Autodesk Fusion 360 part; units mm, degrees
(part 2 of 2)
  spline S17 degree 5 poles (16.2711, -4.6208) (16.2922, -4.6268) (16.3347, -4.6379) (16.399, -4.6517) (16.4857, -4.6647) (16.5954, -4.6738) (16.706, -4.6779) (16.8173, -4.6789) (16.9288, -4.6784) (17.0405, -4.6766) (17.1524, -4.6734) (17.2646, -4.6683) (17.377, -4.6608) (17.4898, -4.6505) (17.6029, -4.6377) (17.7161, -4.6224) (17.8296, -4.6052) (17.9431, -4.5863) (18.0567, -4.5658) (18.1703, -4.5438) (18.284, -4.5203) (18.3977, -4.4951) (18.5115, -4.4682) (18.6252, -4.4395) (18.739, -4.4092) (18.8527, -4.3772) (18.9664, -4.3437) (19.08, -4.3087) (19.1936, -4.2723) (19.3071, -4.2345) (19.4204, -4.1952) (19.5337, -4.1545) (19.6469, -4.1124) (19.7599, -4.0688) (19.8727, -4.0239) (19.9855, -3.9776) (20.098, -3.9299) (20.2104, -3.8809) (20.3225, -3.8306) (20.4345, -3.779) (20.5463, -3.7261) (20.6578, -3.6719) (20.7692, -3.6164) (20.8802, -3.5597) (20.9911, -3.5017) (21.1017, -3.4425) (21.212, -3.3821) (21.322, -3.3204) (21.4317, -3.2575) (21.5412, -3.1935) (21.6503, -3.1282) (21.7592, -3.0618) (21.8677, -2.9942) (21.9759, -2.9255) (22.0837, -2.8556) (22.1912, -2.7845) (22.2984, -2.7123) (22.4052, -2.639) (22.5116, -2.5646) (22.6176, -2.4891) (22.7233, -2.4125) (22.8286, -2.3348) (22.9335, -2.256) (23.0379, -2.1761) (23.142, -2.0952) (23.2456, -2.0132) (23.3488, -1.9301) (23.4516, -1.846) (23.5539, -1.7609) (23.6558, -1.6748) (23.7572, -1.5876) (23.838, -1.517) (23.8983, -1.4636) (23.9385, -1.4279) (23.9586, -1.4099) knots 0 0 0 0 0 0 0.01428571 0.02857143 0.04285714 0.05714286 0.07142857 0.08571429 0.1 0.11428571 0.12857143 0.14285714 0.15714286 0.17142857 0.18571429 0.2 0.21428571 0.22857143 0.24285714 0.25714286 0.27142857 0.28571429 0.3 0.31428571 0.32857143 0.34285714 0.35714286 0.37142857 0.38571429 0.4 0.41428571 0.42857143 0.44285714 0.45714286 0.47142857 0.48571429 0.5 0.51428571 0.52857143 0.54285714 0.55714286 0.57142857 0.58571429 0.6 0.61428571 0.62857143 0.64285714 0.65714286 0.67142857 0.68571429 0.7 0.71428571 0.72857143 0.74285714 0.75714286 0.77142857 0.78571429 0.8 0.81428571 0.82857143 0.84285714 0.85714286 0.87142857 0.88571429 0.9 0.91428571 0.92857143 0.94285714 0.95714286 0.97142857 0.98571429 1 1 1 1 1 1
  spline S18 degree 5 poles (-12.1373, -11.7808) (-12.1531, -11.7961) (-12.1839, -11.8274) (-12.228, -11.8761) (-12.2826, -11.9447) (-12.3454, -12.0351) (-12.4042, -12.1289) (-12.4607, -12.2247) (-12.516, -12.3216) (-12.5703, -12.4192) (-12.6235, -12.5177) (-12.6752, -12.6174) (-12.7249, -12.7185) (-12.7724, -12.8213) (-12.8178, -12.9257) (-12.8612, -13.0314) (-12.903, -13.1383) (-12.9434, -13.2461) (-12.9825, -13.3547) (-13.0203, -13.4641) (-13.0567, -13.5743) (-13.0917, -13.6853) (-13.1253, -13.7973) (-13.1573, -13.9101) (-13.1879, -14.0238) (-13.2171, -14.1383) (-13.245, -14.2535) (-13.2715, -14.3694) (-13.2967, -14.486) (-13.3207, -14.6032) (-13.3434, -14.721) (-13.3648, -14.8394) (-13.3849, -14.9585) (-13.4037, -15.0781) (-13.4212, -15.1983) (-13.4374, -15.3191) (-13.4524, -15.4404) (-13.4661, -15.5622) (-13.4787, -15.6845) (-13.49, -15.8073) (-13.5, -15.9306) (-13.5089, -16.0543) (-13.5165, -16.1784) (-13.5229, -16.303) (-13.5281, -16.4279) (-13.5321, -16.5533) (-13.5349, -16.6791) (-13.5365, -16.8052) (-13.537, -16.9317) (-13.5362, -17.0585) (-13.5343, -17.1856) (-13.5312, -17.3131) (-13.5269, -17.4409) (-13.5215, -17.5689) (-13.5148, -17.6973) (-13.5071, -17.8259) (-13.4981, -17.9548) (-13.4881, -18.0839) (-13.4768, -18.2133) (-13.4644, -18.3429) (-13.4509, -18.4727) (-13.4363, -18.6027) (-13.4205, -18.733) (-13.4035, -18.8634) (-13.3855, -18.994) (-13.3663, -19.1247) (-13.3459, -19.2556) (-13.3245, -19.3866) (-13.3019, -19.5178) (-13.2783, -19.6491) (-13.2535, -19.7805) (-13.2328, -19.8858) (-13.2167, -19.9647) (-13.2058, -20.0174) (-13.2003, -20.0438) knots 0 0 0 0 0 0 0.01428571 0.02857143 0.04285714 0.05714286 0.07142857 0.08571429 0.1 0.11428571 0.12857143 0.14285714 0.15714286 0.17142857 0.18571429 0.2 0.21428571 0.22857143 0.24285714 0.25714286 0.27142857 0.28571429 0.3 0.31428571 0.32857143 0.34285714 0.35714286 0.37142857 0.38571429 0.4 0.41428571 0.42857143 0.44285714 0.45714286 0.47142857 0.48571429 0.5 0.51428571 0.52857143 0.54285714 0.55714286 0.57142857 0.58571429 0.6 0.61428571 0.62857143 0.64285714 0.65714286 0.67142857 0.68571429 0.7 0.71428571 0.72857143 0.74285714 0.75714286 0.77142857 0.78571429 0.8 0.81428571 0.82857143 0.84285714 0.85714286 0.87142857 0.88571429 0.9 0.91428571 0.92857143 0.94285714 0.95714286 0.97142857 0.98571429 1 1 1 1 1 1
  spline S19 degree 5 poles (-13.2003, 20.0438) (-13.2058, 20.0174) (-13.2167, 19.9647) (-13.2328, 19.8858) (-13.2535, 19.7805) (-13.2783, 19.6491) (-13.3019, 19.5178) (-13.3245, 19.3866) (-13.3459, 19.2556) (-13.3663, 19.1247) (-13.3855, 18.994) (-13.4035, 18.8634) (-13.4205, 18.733) (-13.4363, 18.6027) (-13.4509, 18.4727) (-13.4644, 18.3429) (-13.4768, 18.2133) (-13.4881, 18.0839) (-13.4981, 17.9548) (-13.5071, 17.8259) (-13.5148, 17.6973) (-13.5215, 17.5689) (-13.5269, 17.4409) (-13.5312, 17.3131) (-13.5343, 17.1856) (-13.5362, 17.0585) (-13.537, 16.9317) (-13.5365, 16.8052) (-13.5349, 16.6791) (-13.5321, 16.5533) (-13.5281, 16.4279) (-13.5229, 16.303) (-13.5165, 16.1784) (-13.5089, 16.0543) (-13.5, 15.9306) (-13.49, 15.8073) (-13.4787, 15.6845) (-13.4661, 15.5622) (-13.4524, 15.4404) (-13.4374, 15.3191) (-13.4212, 15.1983) (-13.4037, 15.0781) (-13.3849, 14.9585) (-13.3648, 14.8394) (-13.3434, 14.721) (-13.3207, 14.6032) (-13.2967, 14.486) (-13.2715, 14.3694) (-13.245, 14.2535) (-13.2171, 14.1383) (-13.1879, 14.0238) (-13.1573, 13.9101) (-13.1253, 13.7973) (-13.0917, 13.6853) (-13.0567, 13.5743) (-13.0203, 13.4641) (-12.9825, 13.3547) (-12.9434, 13.2461) (-12.903, 13.1383) (-12.8612, 13.0314) (-12.8178, 12.9257) (-12.7724, 12.8213) (-12.7249, 12.7185) (-12.6752, 12.6174) (-12.6235, 12.5177) (-12.5703, 12.4192) (-12.516, 12.3216) (-12.4607, 12.2247) (-12.4042, 12.1289) (-12.3454, 12.0351) (-12.2826, 11.9447) (-12.228, 11.8761) (-12.1839, 11.8274) (-12.1531, 11.7961) (-12.1373, 11.7808) knots -1 -1 -1 -1 -1 -1 -0.98571429 -0.97142857 -0.95714286 -0.94285714 -0.92857143 -0.91428571 -0.9 -0.88571429 -0.87142857 -0.85714286 -0.84285714 -0.82857143 -0.81428571 -0.8 -0.78571429 -0.77142857 -0.75714286 -0.74285714 -0.72857143 -0.71428571 -0.7 -0.68571429 -0.67142857 -0.65714286 -0.64285714 -0.62857143 -0.61428571 -0.6 -0.58571429 -0.57142857 -0.55714286 -0.54285714 -0.52857143 -0.51428571 -0.5 -0.48571429 -0.47142857 -0.45714286 -0.44285714 -0.42857143 -0.41428571 -0.4 -0.38571429 -0.37142857 -0.35714286 -0.34285714 -0.32857143 -0.31428571 -0.3 -0.28571429 -0.27142857 -0.25714286 -0.24285714 -0.22857143 -0.21428571 -0.2 -0.18571429 -0.17142857 -0.15714286 -0.14285714 -0.12857143 -0.11428571 -0.1 -0.08571429 -0.07142857 -0.05714286 -0.04285714 -0.02857143 -0.01428571 0 0 0 0 0 0
  arc A49 (10.7583, -21.4537) -> (13.2003, -20.0438) centre (0, 0) ccw
  arc A50 (-3.1536, 12.5126) -> (-1.0283, 11.0101) centre (-1.2143, 13.0014) ccw
  spline S20 degree 5 poles (4.1338, -16.4016) (4.1392, -16.4229) (4.1508, -16.4652) (4.171, -16.5278) (4.2031, -16.6094) (4.25, -16.709) (4.3019, -16.8068) (4.3566, -16.9036) (4.4128, -16.9999) (4.4702, -17.0958) (4.5289, -17.1911) (4.5894, -17.2857) (4.6521, -17.3793) (4.7174, -17.4719) (4.7851, -17.5634) (4.8549, -17.6538) (4.9266, -17.7435) (4.9997, -17.8323) (5.0742, -17.9205) (5.1501, -18.0079) (5.2273, -18.0946) (5.306, -18.1804) (5.3862, -18.2655) (5.4679, -18.3497) (5.551, -18.433) (5.6356, -18.5155) (5.7214, -18.5972) (5.8085, -18.6782) (5.8969, -18.7583) (5.9864, -18.8377) (6.0771, -18.9162) (6.1689, -18.9939) (6.262, -19.0709) (6.3562, -19.147) (6.4516, -19.2222) (6.548, -19.2967) (6.6456, -19.3703) (6.7442, -19.4431) (6.8439, -19.5151) (6.9446, -19.5863) (7.0463, -19.6567) (7.149, -19.7262) (7.2527, -19.7948) (7.3573, -19.8627) (7.463, -19.9297) (7.5695, -19.9958) (7.677, -20.0611) (7.7854, -20.1256) (7.8948, -20.1892) (8.005, -20.2519) (8.116, -20.3138) (8.228, -20.3749) (8.3408, -20.4351) (8.4544, -20.4944) (8.5689, -20.5528) (8.6842, -20.6104) (8.8002, -20.6671) (8.9171, -20.723) (9.0348, -20.7779) (9.1532, -20.832) (9.2724, -20.8852) (9.3923, -20.9375) (9.513, -20.9889) (9.6344, -21.0395) (9.7565, -21.0891) (9.8794, -21.1379) (10.0029, -21.1857) (10.1271, -21.2327) (10.252, -21.2787) (10.3775, -21.3239) (10.5037, -21.3681) (10.6052, -21.4028) (10.6816, -21.4284) (10.7327, -21.4453) (10.7583, -21.4537) knots 0 0 0 0 0 0 0.01428571 0.02857143 0.04285714 0.05714286 0.07142857 0.08571429 0.1 0.11428571 0.12857143 0.14285714 0.15714286 0.17142857 0.18571429 0.2 0.21428571 0.22857143 0.24285714 0.25714286 0.27142857 0.28571429 0.3 0.31428571 0.32857143 0.34285714 0.35714286 0.37142857 0.38571429 0.4 0.41428571 0.42857143 0.44285714 0.45714286 0.47142857 0.48571429 0.5 0.51428571 0.52857143 0.54285714 0.55714286 0.57142857 0.58571429 0.6 0.61428571 0.62857143 0.64285714 0.65714286 0.67142857 0.68571429 0.7 0.71428571 0.72857143 0.74285714 0.75714286 0.77142857 0.78571429 0.8 0.81428571 0.82857143 0.84285714 0.85714286 0.87142857 0.88571429 0.9 0.91428571 0.92857143 0.94285714 0.95714286 0.97142857 0.98571429 1 1 1 1 1 1
  spline S21 degree 5 poles (-23.9586, -1.4099) (-23.9385, -1.4279) (-23.8983, -1.4636) (-23.838, -1.517) (-23.7572, -1.5876) (-23.6558, -1.6748) (-23.5539, -1.7609) (-23.4516, -1.846) (-23.3488, -1.9301) (-23.2456, -2.0132) (-23.142, -2.0952) (-23.0379, -2.1761) (-22.9335, -2.256) (-22.8286, -2.3348) (-22.7233, -2.4125) (-22.6176, -2.4891) (-22.5116, -2.5646) (-22.4052, -2.639) (-22.2984, -2.7123) (-22.1912, -2.7845) (-22.0837, -2.8556) (-21.9759, -2.9255) (-21.8677, -2.9942) (-21.7592, -3.0618) (-21.6503, -3.1282) (-21.5412, -3.1935) (-21.4317, -3.2575) (-21.322, -3.3204) (-21.212, -3.3821) (-21.1017, -3.4425) (-20.9911, -3.5017) (-20.8802, -3.5597) (-20.7692, -3.6164) (-20.6578, -3.6719) (-20.5463, -3.7261) (-20.4345, -3.779) (-20.3225, -3.8306) (-20.2104, -3.8809) (-20.098, -3.9299) (-19.9855, -3.9776) (-19.8727, -4.0239) (-19.7599, -4.0688) (-19.6469, -4.1124) (-19.5337, -4.1545) (-19.4204, -4.1952) (-19.3071, -4.2345) (-19.1936, -4.2723) (-19.08, -4.3087) (-18.9664, -4.3437) (-18.8527, -4.3772) (-18.739, -4.4092) (-18.6252, -4.4395) (-18.5115, -4.4682) (-18.3977, -4.4951) (-18.284, -4.5203) (-18.1703, -4.5438) (-18.0567, -4.5658) (-17.9431, -4.5863) (-17.8296, -4.6052) (-17.7161, -4.6224) (-17.6029, -4.6377) (-17.4898, -4.6505) (-17.377, -4.6608) (-17.2646, -4.6683) (-17.1524, -4.6734) (-17.0405, -4.6766) (-16.9288, -4.6784) (-16.8173, -4.6789) (-16.706, -4.6779) (-16.5954, -4.6738) (-16.4857, -4.6647) (-16.399, -4.6517) (-16.3347, -4.6379) (-16.2922, -4.6268) (-16.2711, -4.6208) knots -1 -1 -1 -1 -1 -1 -0.98571429 -0.97142857 -0.95714286 -0.94285714 -0.92857143 -0.91428571 -0.9 -0.88571429 -0.87142857 -0.85714286 -0.84285714 -0.82857143 -0.81428571 -0.8 -0.78571429 -0.77142857 -0.75714286 -0.74285714 -0.72857143 -0.71428571 -0.7 -0.68571429 -0.67142857 -0.65714286 -0.64285714 -0.62857143 -0.61428571 -0.6 -0.58571429 -0.57142857 -0.55714286 -0.54285714 -0.52857143 -0.51428571 -0.5 -0.48571429 -0.47142857 -0.45714286 -0.44285714 -0.42857143 -0.41428571 -0.4 -0.38571429 -0.37142857 -0.35714286 -0.34285714 -0.32857143 -0.31428571 -0.3 -0.28571429 -0.27142857 -0.25714286 -0.24285714 -0.22857143 -0.21428571 -0.2 -0.18571429 -0.17142857 -0.15714286 -0.14285714 -0.12857143 -0.11428571 -0.1 -0.08571429 -0.07142857 -0.05714286 -0.04285714 -0.02857143 -0.01428571 0 0 0 0 0 0
  spline S22 degree 5 poles (-4.1338, 16.4016) (-4.1392, 16.4229) (-4.1508, 16.4652) (-4.171, 16.5278) (-4.2031, 16.6094) (-4.25, 16.709) (-4.3019, 16.8068) (-4.3566, 16.9036) (-4.4128, 16.9999) (-4.4702, 17.0958) (-4.5289, 17.1911) (-4.5894, 17.2857) (-4.6521, 17.3793) (-4.7174, 17.4719) (-4.7851, 17.5634) (-4.8549, 17.6538) (-4.9266, 17.7435) (-4.9997, 17.8323) (-5.0742, 17.9205) (-5.1501, 18.0079) (-5.2273, 18.0946) (-5.306, 18.1804) (-5.3862, 18.2655) (-5.4679, 18.3497) (-5.551, 18.433) (-5.6356, 18.5155) (-5.7214, 18.5972) (-5.8085, 18.6782) (-5.8969, 18.7583) (-5.9864, 18.8377) (-6.0771, 18.9162) (-6.1689, 18.9939) (-6.262, 19.0709) (-6.3562, 19.147) (-6.4516, 19.2222) (-6.548, 19.2967) (-6.6456, 19.3703) (-6.7442, 19.4431) (-6.8439, 19.5151) (-6.9446, 19.5863) (-7.0463, 19.6567) (-7.149, 19.7262) (-7.2527, 19.7948) (-7.3573, 19.8627) (-7.463, 19.9297) (-7.5695, 19.9958) (-7.677, 20.0611) (-7.7854, 20.1256) (-7.8948, 20.1892) (-8.005, 20.2519) (-8.116, 20.3138) (-8.228, 20.3749) (-8.3408, 20.4351) (-8.4544, 20.4944) (-8.5689, 20.5528) (-8.6842, 20.6104) (-8.8002, 20.6671) (-8.9171, 20.723) (-9.0348, 20.7779) (-9.1532, 20.832) (-9.2724, 20.8852) (-9.3923, 20.9375) (-9.513, 20.9889) (-9.6344, 21.0395) (-9.7565, 21.0891) (-9.8794, 21.1379) (-10.0029, 21.1857) (-10.1271, 21.2327) (-10.252, 21.2787) (-10.3775, 21.3239) (-10.5037, 21.3681) (-10.6052, 21.4028) (-10.6816, 21.4284) (-10.7327, 21.4453) (-10.7583, 21.4537) knots 0 0 0 0 0 0 0.01428571 0.02857143 0.04285714 0.05714286 0.07142857 0.08571429 0.1 0.11428571 0.12857143 0.14285714 0.15714286 0.17142857 0.18571429 0.2 0.21428571 0.22857143 0.24285714 0.25714286 0.27142857 0.28571429 0.3 0.31428571 0.32857143 0.34285714 0.35714286 0.37142857 0.38571429 0.4 0.41428571 0.42857143 0.44285714 0.45714286 0.47142857 0.48571429 0.5 0.51428571 0.52857143 0.54285714 0.55714286 0.57142857 0.58571429 0.6 0.61428571 0.62857143 0.64285714 0.65714286 0.67142857 0.68571429 0.7 0.71428571 0.72857143 0.74285714 0.75714286 0.77142857 0.78571429 0.8 0.81428571 0.82857143 0.84285714 0.85714286 0.87142857 0.88571429 0.9 0.91428571 0.92857143 0.94285714 0.95714286 0.97142857 0.98571429 1 1 1 1 1 1
  line L23 (12.4131, -3.5252) -> (16.2711, -4.6208)
  spline S23 degree 5 poles (-16.2711, 4.6208) (-16.2922, 4.6268) (-16.3347, 4.6379) (-16.399, 4.6517) (-16.4857, 4.6647) (-16.5954, 4.6738) (-16.706, 4.6779) (-16.8173, 4.6789) (-16.9288, 4.6784) (-17.0405, 4.6766) (-17.1524, 4.6734) (-17.2646, 4.6683) (-17.377, 4.6608) (-17.4898, 4.6505) (-17.6029, 4.6377) (-17.7161, 4.6224) (-17.8296, 4.6052) (-17.9431, 4.5863) (-18.0567, 4.5658) (-18.1703, 4.5438) (-18.284, 4.5203) (-18.3977, 4.4951) (-18.5115, 4.4682) (-18.6252, 4.4395) (-18.739, 4.4092) (-18.8527, 4.3772) (-18.9664, 4.3437) (-19.08, 4.3087) (-19.1936, 4.2723) (-19.3071, 4.2345) (-19.4204, 4.1952) (-19.5337, 4.1545) (-19.6469, 4.1124) (-19.7599, 4.0688) (-19.8727, 4.0239) (-19.9855, 3.9776) (-20.098, 3.9299) (-20.2104, 3.8809) (-20.3225, 3.8306) (-20.4345, 3.779) (-20.5463, 3.7261) (-20.6578, 3.6719) (-20.7692, 3.6164) (-20.8802, 3.5597) (-20.9911, 3.5017) (-21.1017, 3.4425) (-21.212, 3.3821) (-21.322, 3.3204) (-21.4317, 3.2575) (-21.5412, 3.1935) (-21.6503, 3.1282) (-21.7592, 3.0618) (-21.8677, 2.9942) (-21.9759, 2.9255) (-22.0837, 2.8556) (-22.1912, 2.7845) (-22.2984, 2.7123) (-22.4052, 2.639) (-22.5116, 2.5646) (-22.6176, 2.4891) (-22.7233, 2.4125) (-22.8286, 2.3348) (-22.9335, 2.256) (-23.0379, 2.1761) (-23.142, 2.0952) (-23.2456, 2.0132) (-23.3488, 1.9301) (-23.4516, 1.846) (-23.5539, 1.7609) (-23.6558, 1.6748) (-23.7572, 1.5876) (-23.838, 1.517) (-23.8983, 1.4636) (-23.9385, 1.4279) (-23.9586, 1.4099) knots 0 0 0 0 0 0 0.01428571 0.02857143 0.04285714 0.05714286 0.07142857 0.08571429 0.1 0.11428571 0.12857143 0.14285714 0.15714286 0.17142857 0.18571429 0.2 0.21428571 0.22857143 0.24285714 0.25714286 0.27142857 0.28571429 0.3 0.31428571 0.32857143 0.34285714 0.35714286 0.37142857 0.38571429 0.4 0.41428571 0.42857143 0.44285714 0.45714286 0.47142857 0.48571429 0.5 0.51428571 0.52857143 0.54285714 0.55714286 0.57142857 0.58571429 0.6 0.61428571 0.62857143 0.64285714 0.65714286 0.67142857 0.68571429 0.7 0.71428571 0.72857143 0.74285714 0.75714286 0.77142857 0.78571429 0.8 0.81428571 0.82857143 0.84285714 0.85714286 0.87142857 0.88571429 0.9 0.91428571 0.92857143 0.94285714 0.95714286 0.97142857 0.98571429 1 1 1 1 1 1
  arc A51 (9.0209, -6.3956) -> (9.2594, -8.9875) centre (10.6524, -7.5523) ccw
  arc A52 (-1.0283, -11.0101) -> (1.0283, -11.0101) centre (0, 0) ccw
extrude "Extrude3" add sketch "Spacer and Cap" along normal blind 4.2 separate body contours A24 A34 | A36 makes body 2
extrude "Extrude4" add sketch "Spacer and Cap" along normal blind 4.2 separate body contours A37 makes body 3
extrude "Extrude5" add 1 faces at (-8.6071, 0.7949, 8.4) along direction (0, 0, 1) blind 4.2 separate body on bodies 3 makes body 4
sketch "Motor attachment piece" plane through (0, 0, 12.6) normal (0, 0, 1) x (-1, 0, 0)
  circle A0 centre (0, 0) radius 10
  circle A1 centre (0, 0) radius 10
  circle A2 centre (0, 0) radius 2.7
  line L0 (1.85, -4) -> (-1.85, -4)
  line L1 (-1.85, -4) -> (-1.85, 4)
  line L2 (-1.85, 4) -> (1.85, 4)
  line L3 (1.85, 4) -> (1.85, -4)
  line L4 (1.85, -4) -> (-1.85, 4) construction
  line L5 (-1.85, -4) -> (1.85, 4) construction
  dimension "d16" = 5.4
  dimension "d17" = 3.7
  dimension "d18" = 8
  constraint horizontal L0
  constraint perpendicular L0 L1
  constraint parallel L0 L2
  constraint parallel L1 L3
  constraint coincident L4 A0.centre
  constraint coincident L5 A0.centre
  constraint coincident A0.centre A1.centre
  measures "d16" diameter of A2
  measures "d17" distance of L1.end L2.end
  measures "d18" distance of L0.end L1.end
extrude "Extrude6" add sketch "Motor attachment piece" along normal blind 4.2 separate body contours A0 A1 | A2 L3 | A2 L1 L2 L3 | A2 L0 L1 L3 | A2 L1 makes body 5
copy_body "CopyPasteBodies1" bodies 2 makes body 6
move_body "Move1" bodies 6 to x (1, 0, 0) y (0, 1, 0) z (0, 0, 1) at (-37.381, -1.1074, 0)
sketch "Back Cap" plane through (0, 0, 8.4) normal (0, 0, 1) x (-1, 0, 0)
  circle A0 centre (37.381, 1.1074) radius 3.25
  circle A1 centre (37.381, 1.1074) radius 6
  dimension "d23" = 12
  constraint concentric A0 A1
  measures "d23" diameter of A1
extrude "Extrude8" add sketch "Back Cap" against normal blind 4.2 bodies 6
move_body "Move2" bodies 3 to x (1, 0, 0) y (0, 1, 0) z (0, 0, 1) at (45.3922, 3.4121, 0)
move_body "Move3" bodies 4 to x (1, 0, 0) y (0, 1, 0) z (0, 0, 1) at (31.6318, -22.3587, 0)
move_body "Move4" bodies 2 to x (1, 0, 0) y (0, 1, 0) z (0, 0, 1) at (34.427, 25.1789, 0)
move_body "Move5" bodies 5 to x (1, 0, 0) y (0, 1, 0) z (0, 0, 1) at (-28.8671, -19.0156, 0)
move_body "Move6" bodies 3 to x (1, 0, 0) y (0, 1, 0) z (0, 0, 1) at (-76.3852, 16.0977, 0)
move_body "Move7" bodies 4 to x (1, 0, 0) y (0, 1, 0) z (0, 0, 1) at (-36.2987, 58.8671, 0)
move_body "Move8" bodies 2 to x (1, 0, 0) y (0, 1, 0) z (0, 0, 1) at (-56.0263, 8.838, 0)
sketch "For Cutting" plane through (0, 0, 0) normal (0, 0, 1) x (1, 0, 0)
  arc A0 (9.0209, -6.3956) -> (10.0492, -4.6145) centre (0, 0) ccw
  arc A1 (12.4131, -3.5252) -> (10.0492, -4.6145) centre (11.8667, -5.4491) ccw
  line L0 (12.4131, -3.5252) -> (16.2711, -4.6208)
  spline S0 degree 5 poles (16.2711, -4.6208) (16.2922, -4.6268) (16.3347, -4.6379) (16.399, -4.6517) (16.4857, -4.6647) (16.5954, -4.6738) (16.706, -4.6779) (16.8173, -4.6789) (16.9288, -4.6784) (17.0405, -4.6766) (17.1524, -4.6734) (17.2646, -4.6683) (17.377, -4.6608) (17.4898, -4.6505) (17.6029, -4.6377) (17.7161, -4.6224) (17.8296, -4.6052) (17.9431, -4.5863) (18.0567, -4.5658) (18.1703, -4.5438) (18.284, -4.5203) (18.3977, -4.4951) (18.5115, -4.4682) (18.6252, -4.4395) (18.739, -4.4092) (18.8527, -4.3772) (18.9664, -4.3437) (19.08, -4.3087) (19.1936, -4.2723) (19.3071, -4.2345) (19.4204, -4.1952) (19.5337, -4.1545) (19.6469, -4.1124) (19.7599, -4.0688) (19.8727, -4.0239) (19.9855, -3.9776) (20.098, -3.9299) (20.2104, -3.8809) (20.3225, -3.8306) (20.4345, -3.779) (20.5463, -3.7261) (20.6578, -3.6719) (20.7692, -3.6164) (20.8802, -3.5597) (20.9911, -3.5017) (21.1017, -3.4425) (21.212, -3.3821) (21.322, -3.3204) (21.4317, -3.2575) (21.5412, -3.1935) (21.6503, -3.1282) (21.7592, -3.0618) (21.8677, -2.9942) (21.9759, -2.9255) (22.0837, -2.8556) (22.1912, -2.7845) (22.2984, -2.7123) (22.4052, -2.639) (22.5116, -2.5646) (22.6176, -2.4891) (22.7233, -2.4125) (22.8286, -2.3348) (22.9335, -2.256) (23.0379, -2.1761) (23.142, -2.0952) (23.2456, -2.0132) (23.3488, -1.9301) (23.4516, -1.846) (23.5539, -1.7609) (23.6558, -1.6748) (23.7572, -1.5876) (23.838, -1.517) (23.8983, -1.4636) (23.9385, -1.4279) (23.9586, -1.4099) knots 0 0 0 0 0 0 0.01428571 0.02857143 0.04285714 0.05714286 0.07142857 0.08571429 0.1 0.11428571 0.12857143 0.14285714 0.15714286 0.17142857 0.18571429 0.2 0.21428571 0.22857143 0.24285714 0.25714286 0.27142857 0.28571429 0.3 0.31428571 0.32857143 0.34285714 0.35714286 0.37142857 0.38571429 0.4 0.41428571 0.42857143 0.44285714 0.45714286 0.47142857 0.48571429 0.5 0.51428571 0.52857143 0.54285714 0.55714286 0.57142857 0.58571429 0.6 0.61428571 0.62857143 0.64285714 0.65714286 0.67142857 0.68571429 0.7 0.71428571 0.72857143 0.74285714 0.75714286 0.77142857 0.78571429 0.8 0.81428571 0.82857143 0.84285714 0.85714286 0.87142857 0.88571429 0.9 0.91428571 0.92857143 0.94285714 0.95714286 0.97142857 0.98571429 1 1 1 1 1 1
  arc A2 (23.9586, -1.4099) -> (23.9586, 1.4099) centre (0, 0) ccw
  spline S1 degree 5 poles (23.9586, 1.4099) (23.9385, 1.4279) (23.8983, 1.4636) (23.838, 1.517) (23.7572, 1.5876) (23.6558, 1.6748) (23.5539, 1.7609) (23.4516, 1.846) (23.3488, 1.9301) (23.2456, 2.0132) (23.142, 2.0952) (23.0379, 2.1761) (22.9335, 2.256) (22.8286, 2.3348) (22.7233, 2.4125) (22.6176, 2.4891) (22.5116, 2.5646) (22.4052, 2.639) (22.2984, 2.7123) (22.1912, 2.7845) (22.0837, 2.8556) (21.9759, 2.9255) (21.8677, 2.9942) (21.7592, 3.0618) (21.6503, 3.1282) (21.5412, 3.1935) (21.4317, 3.2575) (21.322, 3.3204) (21.212, 3.3821) (21.1017, 3.4425) (20.9911, 3.5017) (20.8802, 3.5597) (20.7692, 3.6164) (20.6578, 3.6719) (20.5463, 3.7261) (20.4345, 3.779) (20.3225, 3.8306) (20.2104, 3.8809) (20.098, 3.9299) (19.9855, 3.9776) (19.8727, 4.0239) (19.7599, 4.0688) (19.6469, 4.1124) (19.5337, 4.1545) (19.4204, 4.1952) (19.3071, 4.2345) (19.1936, 4.2723) (19.08, 4.3087) (18.9664, 4.3437) (18.8527, 4.3772) (18.739, 4.4092) (18.6252, 4.4395) (18.5115, 4.4682) (18.3977, 4.4951) (18.284, 4.5203) (18.1703, 4.5438) (18.0567, 4.5658) (17.9431, 4.5863) (17.8296, 4.6052) (17.7161, 4.6224) (17.6029, 4.6377) (17.4898, 4.6505) (17.377, 4.6608) (17.2646, 4.6683) (17.1524, 4.6734) (17.0405, 4.6766) (16.9288, 4.6784) (16.8173, 4.6789) (16.706, 4.6779) (16.5954, 4.6738) (16.4857, 4.6647) (16.399, 4.6517) (16.3347, 4.6379) (16.2922, 4.6268) (16.2711, 4.6208) knots -1 -1 -1 -1 -1 -1 -0.98571429 -0.97142857 -0.95714286 -0.94285714 -0.92857143 -0.91428571 -0.9 -0.88571429 -0.87142857 -0.85714286 -0.84285714 -0.82857143 -0.81428571 -0.8 -0.78571429 -0.77142857 -0.75714286 -0.74285714 -0.72857143 -0.71428571 -0.7 -0.68571429 -0.67142857 -0.65714286 -0.64285714 -0.62857143 -0.61428571 -0.6 -0.58571429 -0.57142857 -0.55714286 -0.54285714 -0.52857143 -0.51428571 -0.5 -0.48571429 -0.47142857 -0.45714286 -0.44285714 -0.42857143 -0.41428571 -0.4 -0.38571429 -0.37142857 -0.35714286 -0.34285714 -0.32857143 -0.31428571 -0.3 -0.28571429 -0.27142857 -0.25714286 -0.24285714 -0.22857143 -0.21428571 -0.2 -0.18571429 -0.17142857 -0.15714286 -0.14285714 -0.12857143 -0.11428571 -0.1 -0.08571429 -0.07142857 -0.05714286 -0.04285714 -0.02857143 -0.01428571 0 0 0 0 0 0
  line L1 (16.2711, 4.6208) -> (12.4131, 3.5252)
  arc A3 (10.0492, 4.6145) -> (12.4131, 3.5252) centre (11.8667, 5.4491) ccw
  arc A4 (10.0492, 4.6145) -> (9.0209, 6.3956) centre (0, 0) ccw
  arc A5 (9.2594, 8.9875) -> (9.0209, 6.3956) centre (10.6524, 7.5523) ccw
  line L2 (9.2594, 8.9875) -> (12.1373, 11.7808)
  spline S2 degree 5 poles (12.1373, 11.7808) (12.1531, 11.7961) (12.1839, 11.8274) (12.228, 11.8761) (12.2826, 11.9447) (12.3454, 12.0351) (12.4042, 12.1289) (12.4607, 12.2247) (12.516, 12.3216) (12.5703, 12.4192) (12.6235, 12.5177) (12.6752, 12.6174) (12.7249, 12.7185) (12.7724, 12.8213) (12.8178, 12.9257) (12.8612, 13.0314) (12.903, 13.1383) (12.9434, 13.2461) (12.9825, 13.3547) (13.0203, 13.4641) (13.0567, 13.5743) (13.0917, 13.6853) (13.1253, 13.7973) (13.1573, 13.9101) (13.1879, 14.0238) (13.2171, 14.1383) (13.245, 14.2535) (13.2715, 14.3694) (13.2967, 14.486) (13.3207, 14.6032) (13.3434, 14.721) (13.3648, 14.8394) (13.3849, 14.9585) (13.4037, 15.0781) (13.4212, 15.1983) (13.4374, 15.3191) (13.4524, 15.4404) (13.4661, 15.5622) (13.4787, 15.6845) (13.49, 15.8073) (13.5, 15.9306) (13.5089, 16.0543) (13.5165, 16.1784) (13.5229, 16.303) (13.5281, 16.4279) (13.5321, 16.5533) (13.5349, 16.6791) (13.5365, 16.8052) (13.537, 16.9317) (13.5362, 17.0585) (13.5343, 17.1856) (13.5312, 17.3131) (13.5269, 17.4409) (13.5215, 17.5689) (13.5148, 17.6973) (13.5071, 17.8259) (13.4981, 17.9548) (13.4881, 18.0839) (13.4768, 18.2133) (13.4644, 18.3429) (13.4509, 18.4727) (13.4363, 18.6027) (13.4205, 18.733) (13.4035, 18.8634) (13.3855, 18.994) (13.3663, 19.1247) (13.3459, 19.2556) (13.3245, 19.3866) (13.3019, 19.5178) (13.2783, 19.6491) (13.2535, 19.7805) (13.2328, 19.8858) (13.2167, 19.9647) (13.2058, 20.0174) (13.2003, 20.0438) knots 0 0 0 0 0 0 0.01428571 0.02857143 0.04285714 0.05714286 0.07142857 0.08571429 0.1 0.11428571 0.12857143 0.14285714 0.15714286 0.17142857 0.18571429 0.2 0.21428571 0.22857143 0.24285714 0.25714286 0.27142857 0.28571429 0.3 0.31428571 0.32857143 0.34285714 0.35714286 0.37142857 0.38571429 0.4 0.41428571 0.42857143 0.44285714 0.45714286 0.47142857 0.48571429 0.5 0.51428571 0.52857143 0.54285714 0.55714286 0.57142857 0.58571429 0.6 0.61428571 0.62857143 0.64285714 0.65714286 0.67142857 0.68571429 0.7 0.71428571 0.72857143 0.74285714 0.75714286 0.77142857 0.78571429 0.8 0.81428571 0.82857143 0.84285714 0.85714286 0.87142857 0.88571429 0.9 0.91428571 0.92857143 0.94285714 0.95714286 0.97142857 0.98571429 1 1 1 1 1 1
  arc A6 (13.2003, 20.0438) -> (10.7583, 21.4537) centre (0, 0) ccw
  spline S3 degree 5 poles (10.7583, 21.4537) (10.7327, 21.4453) (10.6816, 21.4284) (10.6052, 21.4028) (10.5037, 21.3681) (10.3775, 21.3239) (10.252, 21.2787) (10.1271, 21.2327) (10.0029, 21.1857) (9.8794, 21.1379) (9.7565, 21.0891) (9.6344, 21.0395) (9.513, 20.9889) (9.3923, 20.9375) (9.2724, 20.8852) (9.1532, 20.832) (9.0348, 20.7779) (8.9171, 20.723) (8.8002, 20.6671) (8.6842, 20.6104) (8.5689, 20.5528) (8.4544, 20.4944) (8.3408, 20.4351) (8.228, 20.3749) (8.116, 20.3138) (8.005, 20.2519) (7.8948, 20.1892) (7.7854, 20.1256) (7.677, 20.0611) (7.5695, 19.9958) (7.463, 19.9297) (7.3573, 19.8627) (7.2527, 19.7948) (7.149, 19.7262) (7.0463, 19.6567) (6.9446, 19.5863) (6.8439, 19.5151) (6.7442, 19.4431) (6.6456, 19.3703) (6.548, 19.2967) (6.4516, 19.2222) (6.3562, 19.147) (6.262, 19.0709) (6.1689, 18.9939) (6.0771, 18.9162) (5.9864, 18.8377) (5.8969, 18.7583) (5.8085, 18.6782) (5.7214, 18.5972) (5.6356, 18.5155) (5.551, 18.433) (5.4679, 18.3497) (5.3862, 18.2655) (5.306, 18.1804) (5.2273, 18.0946) (5.1501, 18.0079) (5.0742, 17.9205) (4.9997, 17.8323) (4.9266, 17.7435) (4.8549, 17.6538) (4.7851, 17.5634) (4.7174, 17.4719) (4.6521, 17.3793) (4.5894, 17.2857) (4.5289, 17.1911) (4.4702, 17.0958) (4.4128, 16.9999) (4.3566, 16.9036) (4.3019, 16.8068) (4.25, 16.709) (4.2031, 16.6094) (4.171, 16.5278) (4.1508, 16.4652) (4.1392, 16.4229) (4.1338, 16.4016) knots -1 -1 -1 -1 -1 -1 -0.98571429 -0.97142857 -0.95714286 -0.94285714 -0.92857143 -0.91428571 -0.9 -0.88571429 -0.87142857 -0.85714286 -0.84285714 -0.82857143 -0.81428571 -0.8 -0.78571429 -0.77142857 -0.75714286 -0.74285714 -0.72857143 -0.71428571 -0.7 -0.68571429 -0.67142857 -0.65714286 -0.64285714 -0.62857143 -0.61428571 -0.6 -0.58571429 -0.57142857 -0.55714286 -0.54285714 -0.52857143 -0.51428571 -0.5 -0.48571429 -0.47142857 -0.45714286 -0.44285714 -0.42857143 -0.41428571 -0.4 -0.38571429 -0.37142857 -0.35714286 -0.34285714 -0.32857143 -0.31428571 -0.3 -0.28571429 -0.27142857 -0.25714286 -0.24285714 -0.22857143 -0.21428571 -0.2 -0.18571429 -0.17142857 -0.15714286 -0.14285714 -0.12857143 -0.11428571 -0.1 -0.08571429 -0.07142857 -0.05714286 -0.04285714 -0.02857143 -0.01428571 0 0 0 0 0 0
  line L3 (4.1338, 16.4016) -> (3.1536, 12.5126)
  arc A7 (1.0283, 11.0101) -> (3.1536, 12.5126) centre (1.2143, 13.0014) ccw
  arc A8 (1.0283, 11.0101) -> (-1.0283, 11.0101) centre (0, 0) ccw
  arc A9 (-3.1536, 12.5126) -> (-1.0283, 11.0101) centre (-1.2143, 13.0014) ccw
  line L4 (-3.1536, 12.5126) -> (-4.1338, 16.4016)
  spline S4 degree 5 poles (-4.1338, 16.4016) (-4.1392, 16.4229) (-4.1508, 16.4652) (-4.171, 16.5278) (-4.2031, 16.6094) (-4.25, 16.709) (-4.3019, 16.8068) (-4.3566, 16.9036) (-4.4128, 16.9999) (-4.4702, 17.0958) (-4.5289, 17.1911) (-4.5894, 17.2857) (-4.6521, 17.3793) (-4.7174, 17.4719) (-4.7851, 17.5634) (-4.8549, 17.6538) (-4.9266, 17.7435) (-4.9997, 17.8323) (-5.0742, 17.9205) (-5.1501, 18.0079) (-5.2273, 18.0946) (-5.306, 18.1804) (-5.3862, 18.2655) (-5.4679, 18.3497) (-5.551, 18.433) (-5.6356, 18.5155) (-5.7214, 18.5972) (-5.8085, 18.6782) (-5.8969, 18.7583) (-5.9864, 18.8377) (-6.0771, 18.9162) (-6.1689, 18.9939) (-6.262, 19.0709) (-6.3562, 19.147) (-6.4516, 19.2222) (-6.548, 19.2967) (-6.6456, 19.3703) (-6.7442, 19.4431) (-6.8439, 19.5151) (-6.9446, 19.5863) (-7.0463, 19.6567) (-7.149, 19.7262) (-7.2527, 19.7948) (-7.3573, 19.8627) (-7.463, 19.9297) (-7.5695, 19.9958) (-7.677, 20.0611) (-7.7854, 20.1256) (-7.8948, 20.1892) (-8.005, 20.2519) (-8.116, 20.3138) (-8.228, 20.3749) (-8.3408, 20.4351) (-8.4544, 20.4944) (-8.5689, 20.5528) (-8.6842, 20.6104) (-8.8002, 20.6671) (-8.9171, 20.723) (-9.0348, 20.7779) (-9.1532, 20.832) (-9.2724, 20.8852) (-9.3923, 20.9375) (-9.513, 20.9889) (-9.6344, 21.0395) (-9.7565, 21.0891) (-9.8794, 21.1379) (-10.0029, 21.1857) (-10.1271, 21.2327) (-10.252, 21.2787) (-10.3775, 21.3239) (-10.5037, 21.3681) (-10.6052, 21.4028) (-10.6816, 21.4284) (-10.7327, 21.4453) (-10.7583, 21.4537) knots 0 0 0 0 0 0 0.01428571 0.02857143 0.04285714 0.05714286 0.07142857 0.08571429 0.1 0.11428571 0.12857143 0.14285714 0.15714286 0.17142857 0.18571429 0.2 0.21428571 0.22857143 0.24285714 0.25714286 0.27142857 0.28571429 0.3 0.31428571 0.32857143 0.34285714 0.35714286 0.37142857 0.38571429 0.4 0.41428571 0.42857143 0.44285714 0.45714286 0.47142857 0.48571429 0.5 0.51428571 0.52857143 0.54285714 0.55714286 0.57142857 0.58571429 0.6 0.61428571 0.62857143 0.64285714 0.65714286 0.67142857 0.68571429 0.7 0.71428571 0.72857143 0.74285714 0.75714286 0.77142857 0.78571429 0.8 0.81428571 0.82857143 0.84285714 0.85714286 0.87142857 0.88571429 0.9 0.91428571 0.92857143 0.94285714 0.95714286 0.97142857 0.98571429 1 1 1 1 1 1
  arc A10 (-10.7583, 21.4537) -> (-13.2003, 20.0438) centre (0, 0) ccw
  spline S5 degree 5 poles (-13.2003, 20.0438) (-13.2058, 20.0174) (-13.2167, 19.9647) (-13.2328, 19.8858) (-13.2535, 19.7805) (-13.2783, 19.6491) (-13.3019, 19.5178) (-13.3245, 19.3866) (-13.3459, 19.2556) (-13.3663, 19.1247) (-13.3855, 18.994) (-13.4035, 18.8634) (-13.4205, 18.733) (-13.4363, 18.6027) (-13.4509, 18.4727) (-13.4644, 18.3429) (-13.4768, 18.2133) (-13.4881, 18.0839) (-13.4981, 17.9548) (-13.5071, 17.8259) (-13.5148, 17.6973) (-13.5215, 17.5689) (-13.5269, 17.4409) (-13.5312, 17.3131) (-13.5343, 17.1856) (-13.5362, 17.0585) (-13.537, 16.9317) (-13.5365, 16.8052) (-13.5349, 16.6791) (-13.5321, 16.5533) (-13.5281, 16.4279) (-13.5229, 16.303) (-13.5165, 16.1784) (-13.5089, 16.0543) (-13.5, 15.9306) (-13.49, 15.8073) (-13.4787, 15.6845) (-13.4661, 15.5622) (-13.4524, 15.4404) (-13.4374, 15.3191) (-13.4212, 15.1983) (-13.4037, 15.0781) (-13.3849, 14.9585) (-13.3648, 14.8394) (-13.3434, 14.721) (-13.3207, 14.6032) (-13.2967, 14.486) (-13.2715, 14.3694) (-13.245, 14.2535) (-13.2171, 14.1383) (-13.1879, 14.0238) (-13.1573, 13.9101) (-13.1253, 13.7973) (-13.0917, 13.6853) (-13.0567, 13.5743) (-13.0203, 13.4641) (-12.9825, 13.3547) (-12.9434, 13.2461) (-12.903, 13.1383) (-12.8612, 13.0314) (-12.8178, 12.9257) (-12.7724, 12.8213) (-12.7249, 12.7185) (-12.6752, 12.6174) (-12.6235, 12.5177) (-12.5703, 12.4192) (-12.516, 12.3216) (-12.4607, 12.2247) (-12.4042, 12.1289) (-12.3454, 12.0351) (-12.2826, 11.9447) (-12.228, 11.8761) (-12.1839, 11.8274) (-12.1531, 11.7961) (-12.1373, 11.7808) knots -1 -1 -1 -1 -1 -1 -0.98571429 -0.97142857 -0.95714286 -0.94285714 -0.92857143 -0.91428571 -0.9 -0.88571429 -0.87142857 -0.85714286 -0.84285714 -0.82857143 -0.81428571 -0.8 -0.78571429 -0.77142857 -0.75714286 -0.74285714 -0.72857143 -0.71428571 -0.7 -0.68571429 -0.67142857 -0.65714286 -0.64285714 -0.62857143 -0.61428571 -0.6 -0.58571429 -0.57142857 -0.55714286 -0.54285714 -0.52857143 -0.51428571 -0.5 -0.48571429 -0.47142857 -0.45714286 -0.44285714 -0.42857143 -0.41428571 -0.4 -0.38571429 -0.37142857 -0.35714286 -0.34285714 -0.32857143 -0.31428571 -0.3 -0.28571429 -0.27142857 -0.25714286 -0.24285714 -0.22857143 -0.21428571 -0.2 -0.18571429 -0.17142857 -0.15714286 -0.14285714 -0.12857143 -0.11428571 -0.1 -0.08571429 -0.07142857 -0.05714286 -0.04285714 -0.02857143 -0.01428571 0 0 0 0 0 0
  line L5 (-12.1373, 11.7808) -> (-9.2594, 8.9875)
  arc A11 (-9.0209, 6.3956) -> (-9.2594, 8.9875) centre (-10.6524, 7.5523) ccw
  arc A12 (-9.0209, 6.3956) -> (-10.0492, 4.6145) centre (0, 0) ccw
  arc A13 (-12.4131, 3.5252) -> (-10.0492, 4.6145) centre (-11.8667, 5.4491) ccw
  line L6 (-12.4131, 3.5252) -> (-16.2711, 4.6208)
  spline S6 degree 5 poles (-16.2711, 4.6208) (-16.2922, 4.6268) (-16.3347, 4.6379) (-16.399, 4.6517) (-16.4857, 4.6647) (-16.5954, 4.6738) (-16.706, 4.6779) (-16.8173, 4.6789) (-16.9288, 4.6784) (-17.0405, 4.6766) (-17.1524, 4.6734) (-17.2646, 4.6683) (-17.377, 4.6608) (-17.4898, 4.6505) (-17.6029, 4.6377) (-17.7161, 4.6224) (-17.8296, 4.6052) (-17.9431, 4.5863) (-18.0567, 4.5658) (-18.1703, 4.5438) (-18.284, 4.5203) (-18.3977, 4.4951) (-18.5115, 4.4682) (-18.6252, 4.4395) (-18.739, 4.4092) (-18.8527, 4.3772) (-18.9664, 4.3437) (-19.08, 4.3087) (-19.1936, 4.2723) (-19.3071, 4.2345) (-19.4204, 4.1952) (-19.5337, 4.1545) (-19.6469, 4.1124) (-19.7599, 4.0688) (-19.8727, 4.0239) (-19.9855, 3.9776) (-20.098, 3.9299) (-20.2104, 3.8809) (-20.3225, 3.8306) (-20.4345, 3.779) (-20.5463, 3.7261) (-20.6578, 3.6719) (-20.7692, 3.6164) (-20.8802, 3.5597) (-20.9911, 3.5017) (-21.1017, 3.4425) (-21.212, 3.3821) (-21.322, 3.3204) (-21.4317, 3.2575) (-21.5412, 3.1935) (-21.6503, 3.1282) (-21.7592, 3.0618) (-21.8677, 2.9942) (-21.9759, 2.9255) (-22.0837, 2.8556) (-22.1912, 2.7845) (-22.2984, 2.7123) (-22.4052, 2.639) (-22.5116, 2.5646) (-22.6176, 2.4891) (-22.7233, 2.4125) (-22.8286, 2.3348) (-22.9335, 2.256) (-23.0379, 2.1761) (-23.142, 2.0952) (-23.2456, 2.0132) (-23.3488, 1.9301) (-23.4516, 1.846) (-23.5539, 1.7609) (-23.6558, 1.6748) (-23.7572, 1.5876) (-23.838, 1.517) (-23.8983, 1.4636) (-23.9385, 1.4279) (-23.9586, 1.4099) knots 0 0 0 0 0 0 0.01428571 0.02857143 0.04285714 0.05714286 0.07142857 0.08571429 0.1 0.11428571 0.12857143 0.14285714 0.15714286 0.17142857 0.18571429 0.2 0.21428571 0.22857143 0.24285714 0.25714286 0.27142857 0.28571429 0.3 0.31428571 0.32857143 0.34285714 0.35714286 0.37142857 0.38571429 0.4 0.41428571 0.42857143 0.44285714 0.45714286 0.47142857 0.48571429 0.5 0.51428571 0.52857143 0.54285714 0.55714286 0.57142857 0.58571429 0.6 0.61428571 0.62857143 0.64285714 0.65714286 0.67142857 0.68571429 0.7 0.71428571 0.72857143 0.74285714 0.75714286 0.77142857 0.78571429 0.8 0.81428571 0.82857143 0.84285714 0.85714286 0.87142857 0.88571429 0.9 0.91428571 0.92857143 0.94285714 0.95714286 0.97142857 0.98571429 1 1 1 1 1 1
  arc A14 (-23.9586, 1.4099) -> (-23.9586, -1.4099) centre (0, 0) ccw
  spline S7 degree 5 poles (-23.9586, -1.4099) (-23.9385, -1.4279) (-23.8983, -1.4636) (-23.838, -1.517) (-23.7572, -1.5876) (-23.6558, -1.6748) (-23.5539, -1.7609) (-23.4516, -1.846) (-23.3488, -1.9301) (-23.2456, -2.0132) (-23.142, -2.0952) (-23.0379, -2.1761) (-22.9335, -2.256) (-22.8286, -2.3348) (-22.7233, -2.4125) (-22.6176, -2.4891) (-22.5116, -2.5646) (-22.4052, -2.639) (-22.2984, -2.7123) (-22.1912, -2.7845) (-22.0837, -2.8556) (-21.9759, -2.9255) (-21.8677, -2.9942) (-21.7592, -3.0618) (-21.6503, -3.1282) (-21.5412, -3.1935) (-21.4317, -3.2575) (-21.322, -3.3204) (-21.212, -3.3821) (-21.1017, -3.4425) (-20.9911, -3.5017) (-20.8802, -3.5597) (-20.7692, -3.6164) (-20.6578, -3.6719) (-20.5463, -3.7261) (-20.4345, -3.779) (-20.3225, -3.8306) (-20.2104, -3.8809) (-20.098, -3.9299) (-19.9855, -3.9776) (-19.8727, -4.0239) (-19.7599, -4.0688) (-19.6469, -4.1124) (-19.5337, -4.1545) (-19.4204, -4.1952) (-19.3071, -4.2345) (-19.1936, -4.2723) (-19.08, -4.3087) (-18.9664, -4.3437) (-18.8527, -4.3772) (-18.739, -4.4092) (-18.6252, -4.4395) (-18.5115, -4.4682) (-18.3977, -4.4951) (-18.284, -4.5203) (-18.1703, -4.5438) (-18.0567, -4.5658) (-17.9431, -4.5863) (-17.8296, -4.6052) (-17.7161, -4.6224) (-17.6029, -4.6377) (-17.4898, -4.6505) (-17.377, -4.6608) (-17.2646, -4.6683) (-17.1524, -4.6734) (-17.0405, -4.6766) (-16.9288, -4.6784) (-16.8173, -4.6789) (-16.706, -4.6779) (-16.5954, -4.6738) (-16.4857, -4.6647) (-16.399, -4.6517) (-16.3347, -4.6379) (-16.2922, -4.6268) (-16.2711, -4.6208) knots -1 -1 -1 -1 -1 -1 -0.98571429 -0.97142857 -0.95714286 -0.94285714 -0.92857143 -0.91428571 -0.9 -0.88571429 -0.87142857 -0.85714286 -0.84285714 -0.82857143 -0.81428571 -0.8 -0.78571429 -0.77142857 -0.75714286 -0.74285714 -0.72857143 -0.71428571 -0.7 -0.68571429 -0.67142857 -0.65714286 -0.64285714 -0.62857143 -0.61428571 -0.6 -0.58571429 -0.57142857 -0.55714286 -0.54285714 -0.52857143 -0.51428571 -0.5 -0.48571429 -0.47142857 -0.45714286 -0.44285714 -0.42857143 -0.41428571 -0.4 -0.38571429 -0.37142857 -0.35714286 -0.34285714 -0.32857143 -0.31428571 -0.3 -0.28571429 -0.27142857 -0.25714286 -0.24285714 -0.22857143 -0.21428571 -0.2 -0.18571429 -0.17142857 -0.15714286 -0.14285714 -0.12857143 -0.11428571 -0.1 -0.08571429 -0.07142857 -0.05714286 -0.04285714 -0.02857143 -0.01428571 0 0 0 0 0 0
  line L7 (-16.2711, -4.6208) -> (-12.4131, -3.5252)
  arc A15 (-10.0492, -4.6145) -> (-12.4131, -3.5252) centre (-11.8667, -5.4491) ccw
  arc A16 (-10.0492, -4.6145) -> (-9.0209, -6.3956) centre (0, 0) ccw
  arc A17 (-9.2594, -8.9875) -> (-9.0209, -6.3956) centre (-10.6524, -7.5523) ccw
  line L8 (-9.2594, -8.9875) -> (-12.1373, -11.7808)
  spline S8 degree 5 poles (-12.1373, -11.7808) (-12.1531, -11.7961) (-12.1839, -11.8274) (-12.228, -11.8761) (-12.2826, -11.9447) (-12.3454, -12.0351) (-12.4042, -12.1289) (-12.4607, -12.2247) (-12.516, -12.3216) (-12.5703, -12.4192) (-12.6235, -12.5177) (-12.6752, -12.6174) (-12.7249, -12.7185) (-12.7724, -12.8213) (-12.8178, -12.9257) (-12.8612, -13.0314) (-12.903, -13.1383) (-12.9434, -13.2461) (-12.9825, -13.3547) (-13.0203, -13.4641) (-13.0567, -13.5743) (-13.0917, -13.6853) (-13.1253, -13.7973) (-13.1573, -13.9101) (-13.1879, -14.0238) (-13.2171, -14.1383) (-13.245, -14.2535) (-13.2715, -14.3694) (-13.2967, -14.486) (-13.3207, -14.6032) (-13.3434, -14.721) (-13.3648, -14.8394) (-13.3849, -14.9585) (-13.4037, -15.0781) (-13.4212, -15.1983) (-13.4374, -15.3191) (-13.4524, -15.4404) (-13.4661, -15.5622) (-13.4787, -15.6845) (-13.49, -15.8073) (-13.5, -15.9306) (-13.5089, -16.0543) (-13.5165, -16.1784) (-13.5229, -16.303) (-13.5281, -16.4279) (-13.5321, -16.5533) (-13.5349, -16.6791) (-13.5365, -16.8052) (-13.537, -16.9317) (-13.5362, -17.0585) (-13.5343, -17.1856) (-13.5312, -17.3131) (-13.5269, -17.4409) (-13.5215, -17.5689) (-13.5148, -17.6973) (-13.5071, -17.8259) (-13.4981, -17.9548) (-13.4881, -18.0839) (-13.4768, -18.2133) (-13.4644, -18.3429) (-13.4509, -18.4727) (-13.4363, -18.6027) (-13.4205, -18.733) (-13.4035, -18.8634) (-13.3855, -18.994) (-13.3663, -19.1247) (-13.3459, -19.2556) (-13.3245, -19.3866) (-13.3019, -19.5178) (-13.2783, -19.6491) (-13.2535, -19.7805) (-13.2328, -19.8858) (-13.2167, -19.9647) (-13.2058, -20.0174) (-13.2003, -20.0438) knots 0 0 0 0 0 0 0.01428571 0.02857143 0.04285714 0.05714286 0.07142857 0.08571429 0.1 0.11428571 0.12857143 0.14285714 0.15714286 0.17142857 0.18571429 0.2 0.21428571 0.22857143 0.24285714 0.25714286 0.27142857 0.28571429 0.3 0.31428571 0.32857143 0.34285714 0.35714286 0.37142857 0.38571429 0.4 0.41428571 0.42857143 0.44285714 0.45714286 0.47142857 0.48571429 0.5 0.51428571 0.52857143 0.54285714 0.55714286 0.57142857 0.58571429 0.6 0.61428571 0.62857143 0.64285714 0.65714286 0.67142857 0.68571429 0.7 0.71428571 0.72857143 0.74285714 0.75714286 0.77142857 0.78571429 0.8 0.81428571 0.82857143 0.84285714 0.85714286 0.87142857 0.88571429 0.9 0.91428571 0.92857143 0.94285714 0.95714286 0.97142857 0.98571429 1 1 1 1 1 1
  arc A18 (-13.2003, -20.0438) -> (-10.7583, -21.4537) centre (0, 0) ccw
  spline S9 degree 5 poles (-10.7583, -21.4537) (-10.7327, -21.4453) (-10.6816, -21.4284) (-10.6052, -21.4028) (-10.5037, -21.3681) (-10.3775, -21.3239) (-10.252, -21.2787) (-10.1271, -21.2327) (-10.0029, -21.1857) (-9.8794, -21.1379) (-9.7565, -21.0891) (-9.6344, -21.0395) (-9.513, -20.9889) (-9.3923, -20.9375) (-9.2724, -20.8852) (-9.1532, -20.832) (-9.0348, -20.7779) (-8.9171, -20.723) (-8.8002, -20.6671) (-8.6842, -20.6104) (-8.5689, -20.5528) (-8.4544, -20.4944) (-8.3408, -20.4351) (-8.228, -20.3749) (-8.116, -20.3138) (-8.005, -20.2519) (-7.8948, -20.1892) (-7.7854, -20.1256) (-7.677, -20.0611) (-7.5695, -19.9958) (-7.463, -19.9297) (-7.3573, -19.8627) (-7.2527, -19.7948) (-7.149, -19.7262) (-7.0463, -19.6567) (-6.9446, -19.5863) (-6.8439, -19.5151) (-6.7442, -19.4431) (-6.6456, -19.3703) (-6.548, -19.2967) (-6.4516, -19.2222) (-6.3562, -19.147) (-6.262, -19.0709) (-6.1689, -18.9939) (-6.0771, -18.9162) (-5.9864, -18.8377) (-5.8969, -18.7583) (-5.8085, -18.6782) (-5.7214, -18.5972) (-5.6356, -18.5155) (-5.551, -18.433) (-5.4679, -18.3497) (-5.3862, -18.2655) (-5.306, -18.1804) (-5.2273, -18.0946) (-5.1501, -18.0079) (-5.0742, -17.9205) (-4.9997, -17.8323) (-4.9266, -17.7435) (-4.8549, -17.6538) (-4.7851, -17.5634) (-4.7174, -17.4719) (-4.6521, -17.3793) (-4.5894, -17.2857) (-4.5289, -17.1911) (-4.4702, -17.0958) (-4.4128, -16.9999) (-4.3566, -16.9036) (-4.3019, -16.8068) (-4.25, -16.709) (-4.2031, -16.6094) (-4.171, -16.5278) (-4.1508, -16.4652) (-4.1392, -16.4229) (-4.1338, -16.4016) knots -1 -1 -1 -1 -1 -1 -0.98571429 -0.97142857 -0.95714286 -0.94285714 -0.92857143 -0.91428571 -0.9 -0.88571429 -0.87142857 -0.85714286 -0.84285714 -0.82857143 -0.81428571 -0.8 -0.78571429 -0.77142857 -0.75714286 -0.74285714 -0.72857143 -0.71428571 -0.7 -0.68571429 -0.67142857 -0.65714286 -0.64285714 -0.62857143 -0.61428571 -0.6 -0.58571429 -0.57142857 -0.55714286 -0.54285714 -0.52857143 -0.51428571 -0.5 -0.48571429 -0.47142857 -0.45714286 -0.44285714 -0.42857143 -0.41428571 -0.4 -0.38571429 -0.37142857 -0.35714286 -0.34285714 -0.32857143 -0.31428571 -0.3 -0.28571429 -0.27142857 -0.25714286 -0.24285714 -0.22857143 -0.21428571 -0.2 -0.18571429 -0.17142857 -0.15714286 -0.14285714 -0.12857143 -0.11428571 -0.1 -0.08571429 -0.07142857 -0.05714286 -0.04285714 -0.02857143 -0.01428571 0 0 0 0 0 0
  line L9 (-4.1338, -16.4016) -> (-3.1536, -12.5126)
  arc A19 (-1.0283, -11.0101) -> (-3.1536, -12.5126) centre (-1.2143, -13.0014) ccw
  arc A20 (-1.0283, -11.0101) -> (1.0283, -11.0101) centre (0, 0) ccw
  arc A21 (3.1536, -12.5126) -> (1.0283, -11.0101) centre (1.2143, -13.0014) ccw
  line L10 (3.1536, -12.5126) -> (4.1338, -16.4016)
  spline S10 degree 5 poles (4.1338, -16.4016) (4.1392, -16.4229) (4.1508, -16.4652) (4.171, -16.5278) (4.2031, -16.6094) (4.25, -16.709) (4.3019, -16.8068) (4.3566, -16.9036) (4.4128, -16.9999) (4.4702, -17.0958) (4.5289, -17.1911) (4.5894, -17.2857) (4.6521, -17.3793) (4.7174, -17.4719) (4.7851, -17.5634) (4.8549, -17.6538) (4.9266, -17.7435) (4.9997, -17.8323) (5.0742, -17.9205) (5.1501, -18.0079) (5.2273, -18.0946) (5.306, -18.1804) (5.3862, -18.2655) (5.4679, -18.3497) (5.551, -18.433) (5.6356, -18.5155) (5.7214, -18.5972) (5.8085, -18.6782) (5.8969, -18.7583) (5.9864, -18.8377) (6.0771, -18.9162) (6.1689, -18.9939) (6.262, -19.0709) (6.3562, -19.147) (6.4516, -19.2222) (6.548, -19.2967) (6.6456, -19.3703) (6.7442, -19.4431) (6.8439, -19.5151) (6.9446, -19.5863) (7.0463, -19.6567) (7.149, -19.7262) (7.2527, -19.7948) (7.3573, -19.8627) (7.463, -19.9297) (7.5695, -19.9958) (7.677, -20.0611) (7.7854, -20.1256) (7.8948, -20.1892) (8.005, -20.2519) (8.116, -20.3138) (8.228, -20.3749) (8.3408, -20.4351) (8.4544, -20.4944) (8.5689, -20.5528) (8.6842, -20.6104) (8.8002, -20.6671) (8.9171, -20.723) (9.0348, -20.7779) (9.1532, -20.832) (9.2724, -20.8852) (9.3923, -20.9375) (9.513, -20.9889) (9.6344, -21.0395) (9.7565, -21.0891) (9.8794, -21.1379) (10.0029, -21.1857) (10.1271, -21.2327) (10.252, -21.2787) (10.3775, -21.3239) (10.5037, -21.3681) (10.6052, -21.4028) (10.6816, -21.4284) (10.7327, -21.4453) (10.7583, -21.4537) knots 0 0 0 0 0 0 0.01428571 0.02857143 0.04285714 0.05714286 0.07142857 0.08571429 0.1 0.11428571 0.12857143 0.14285714 0.15714286 0.17142857 0.18571429 0.2 0.21428571 0.22857143 0.24285714 0.25714286 0.27142857 0.28571429 0.3 0.31428571 0.32857143 0.34285714 0.35714286 0.37142857 0.38571429 0.4 0.41428571 0.42857143 0.44285714 0.45714286 0.47142857 0.48571429 0.5 0.51428571 0.52857143 0.54285714 0.55714286 0.57142857 0.58571429 0.6 0.61428571 0.62857143 0.64285714 0.65714286 0.67142857 0.68571429 0.7 0.71428571 0.72857143 0.74285714 0.75714286 0.77142857 0.78571429 0.8 0.81428571 0.82857143 0.84285714 0.85714286 0.87142857 0.88571429 0.9 0.91428571 0.92857143 0.94285714 0.95714286 0.97142857 0.98571429 1 1 1 1 1 1
  arc A22 (10.7583, -21.4537) -> (13.2003, -20.0438) centre (0, 0) ccw
  spline S11 degree 5 poles (13.2003, -20.0438) (13.2058, -20.0174) (13.2167, -19.9647) (13.2328, -19.8858) (13.2535, -19.7805) (13.2783, -19.6491) (13.3019, -19.5178) (13.3245, -19.3866) (13.3459, -19.2556) (13.3663, -19.1247) (13.3855, -18.994) (13.4035, -18.8634) (13.4205, -18.733) (13.4363, -18.6027) (13.4509, -18.4727) (13.4644, -18.3429) (13.4768, -18.2133) (13.4881, -18.0839) (13.4981, -17.9548) (13.5071, -17.8259) (13.5148, -17.6973) (13.5215, -17.5689) (13.5269, -17.4409) (13.5312, -17.3131) (13.5343, -17.1856) (13.5362, -17.0585) (13.537, -16.9317) (13.5365, -16.8052) (13.5349, -16.6791) (13.5321, -16.5533) (13.5281, -16.4279) (13.5229, -16.303) (13.5165, -16.1784) (13.5089, -16.0543) (13.5, -15.9306) (13.49, -15.8073) (13.4787, -15.6845) (13.4661, -15.5622) (13.4524, -15.4404) (13.4374, -15.3191) (13.4212, -15.1983) (13.4037, -15.0781) (13.3849, -14.9585) (13.3648, -14.8394) (13.3434, -14.721) (13.3207, -14.6032) (13.2967, -14.486) (13.2715, -14.3694) (13.245, -14.2535) (13.2171, -14.1383) (13.1879, -14.0238) (13.1573, -13.9101) (13.1253, -13.7973) (13.0917, -13.6853) (13.0567, -13.5743) (13.0203, -13.4641) (12.9825, -13.3547) (12.9434, -13.2461) (12.903, -13.1383) (12.8612, -13.0314) (12.8178, -12.9257) (12.7724, -12.8213) (12.7249, -12.7185) (12.6752, -12.6174) (12.6235, -12.5177) (12.5703, -12.4192) (12.516, -12.3216) (12.4607, -12.2247) (12.4042, -12.1289) (12.3454, -12.0351) (12.2826, -11.9447) (12.228, -11.8761) (12.1839, -11.8274) (12.1531, -11.7961) (12.1373, -11.7808) knots -1 -1 -1 -1 -1 -1 -0.98571429 -0.97142857 -0.95714286 -0.94285714 -0.92857143 -0.91428571 -0.9 -0.88571429 -0.87142857 -0.85714286 -0.84285714 -0.82857143 -0.81428571 -0.8 -0.78571429 -0.77142857 -0.75714286 -0.74285714 -0.72857143 -0.71428571 -0.7 -0.68571429 -0.67142857 -0.65714286 -0.64285714 -0.62857143 -0.61428571 -0.6 -0.58571429 -0.57142857 -0.55714286 -0.54285714 -0.52857143 -0.51428571 -0.5 -0.48571429 -0.47142857 -0.45714286 -0.44285714 -0.42857143 -0.41428571 -0.4 -0.38571429 -0.37142857 -0.35714286 -0.34285714 -0.32857143 -0.31428571 -0.3 -0.28571429 -0.27142857 -0.25714286 -0.24285714 -0.22857143 -0.21428571 -0.2 -0.18571429 -0.17142857 -0.15714286 -0.14285714 -0.12857143 -0.11428571 -0.1 -0.08571429 -0.07142857 -0.05714286 -0.04285714 -0.02857143 -0.01428571 0 0 0 0 0 0
  line L11 (12.1373, -11.7808) -> (9.2594, -8.9875)
  arc A23 (9.0209, -6.3956) -> (9.2594, -8.9875) centre (10.6524, -7.5523) ccw
  circle A24 centre (0, 0) radius 2.45
  circle A25 centre (-4.667, 36.5084) radius 6
  circle A26 centre (-4.667, 36.5084) radius 10
  circle A27 centre (-21.5994, 34.0168) radius 3.25
  circle A28 centre (-21.5994, 34.0168) radius 3.25
  circle A29 centre (-30.993, 19.5098) radius 6
  circle A30 centre (-30.993, 19.5098) radius 6
  circle A31 centre (-30.993, 19.5098) radius 10
  circle A32 centre (-37.381, -1.1074) radius 6
  arc A33 (-27.0171, -17.049) -> (-30.7171, -17.049) centre (-28.8671, -19.0156) ccw
  line L12 (-27.0171, -17.049) -> (-27.0171, -20.9822)
  arc A34 (-30.7171, -20.9822) -> (-27.0171, -20.9822) centre (-28.8671, -19.0156) ccw
  line L13 (-30.7171, -20.9822) -> (-30.7171, -17.049)
  circle A35 centre (-28.8671, -19.0156) radius 10
  circle A36 centre (0, 0) radius 6
  circle A37 centre (0, 0) radius 10
equation "thickness = 4.2 mm"
equation "d10 = thickness"
equation "d12 = thickness"
equation "d14 = thickness"
equation "d19 = thickness"
named bodies: "Spur Gear (6 teeth)", "Spacer 1", "Cap", "Spacer 2", "Motor attachment piece", "Back Cap"
